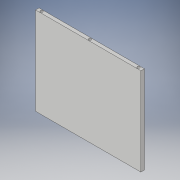
# Autodesk Inventor part: Base
Saved by Autodesk Inventor 2019 (Build 230136000, 136)
## iProperties
Created: 2021-03-05
Part Number: Base
Material: Generic
Document SubType Name: Modeling
Designer: User
Density: 1 g/cm^3
Appearance: Default
Author: User
Autodesk Inventor part; units mm, degrees
ref_plane "YZ Plane" through (0, 0, 0) normal (1, 0, 0) x (0, 1, 0)
ref_plane "XZ Plane" through (0, 0, 0) normal (0, 1, 0) x (-1, 0, 0)
ref_plane "XY Plane" through (0, 0, 0) normal (0, 0, 1) x (1, 0, 0)
sketch "Sketch1" plane through (0, 0, 0) normal (0, 0, 1) x (1, 0, 0)
  line L0 (-137.5, 125) -> (162.5, 125)
  line L1 (162.5, 125) -> (162.5, -125)
  line L2 (162.5, -125) -> (-137.5, -125)
  line L3 (-137.5, -125) -> (-137.5, 125)
  point P0 (0, 0)
  dimension "d0" = 300
  dimension "d1" = 250
  dimension "d2" = 162.5
  dimension "d3" = 125
  constraints: 8 end point, 2 parallel, 1 horizontal, 1 perpendicular
  measures "d0" distance between parallel lines of L1 L3
  measures "d1" distance between parallel lines of L0 L2
  measures "d2" distance from line of L1 point (0, 0)
  measures "d3" distance from line of point (0, 0) L2
extrude "Extrusion1" add sketch "Sketch1" along normal blind 10
sketch "Sketch4" plane through (-137.5, 125, 0) normal (0, 1, 0) x (1, 0, 0)
  circle A0 centre (288, -5) radius 3.5
  circle A1 centre (150, -5) radius 3.5
  circle A2 centre (12, -5) radius 3.5
  line L0 (300, 0) -> (300, -10) projected
  line L1 (0, 0) -> (0, -10) projected
  line L2 (0, 0) -> (300, 0) projected
  point P0 (137.5, 0)
  dimension "d6" = 7
  dimension "d7" = 7
  dimension "d8" = 7
  dimension "d9" = 12
  dimension "d10" = 12
  dimension "d12" = 150
  dimension "d13" = 5
  dimension "d14" = 5
  dimension "d15" = 5
  constraints: 3 centre point
  measures "d6" diameter of A0
  measures "d7" diameter of A1
  measures "d8" diameter of A2
  measures "d9" distance from line of A0.centre L0
  measures "d10" distance from line of L1 A2.centre
  measures "d12" distance from line of A1.centre L0
  measures "d13" distance from line of A0.centre L2
  measures "d14" distance from line of L2 A1.centre
  measures "d15" distance from line of A2.centre L2
extrude "Extrusion2" cut sketch "Sketch4" against normal blind 10
body "Solid1"
